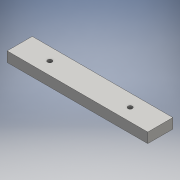
# Autodesk Inventor part: xyStagePostAttach
Saved by Autodesk Inventor 2016 (Build 200138000, 138)
## iProperties
Created: 2016-09-30
Part Number: xyStagePostAttach
Material: Generic
Document SubType Name: Modeling
Designer: sims01
Density: 1 g/cm^3
Appearance: Default
Author: sims01
Autodesk Inventor part; units mm, degrees
ref_plane "YZ Plane" through (0, 0, 0) normal (1, 0, 0) x (0, 1, 0)
ref_plane "XZ Plane" through (0, 0, 0) normal (0, 1, 0) x (-1, 0, 0)
ref_plane "XY Plane" through (0, 0, 0) normal (0, 0, 1) x (1, 0, 0)
sketch "Sketch1" plane through (0, 0, 0) normal (0, 0, 1) x (1, 0, 0)
  line L0 (-70, 12.5) -> (70, 12.5)
  line L1 (70, 12.5) -> (70, -12.5)
  line L2 (70, -12.5) -> (-70, -12.5)
  line L3 (-70, -12.5) -> (-70, 12.5)
  point P0 (0, 0)
  dimension "d0" = 140
  dimension "d1" = 25
  dimension "d2" = 70
  dimension "d3" = 12.5
  constraints: 8 end point, 2 parallel, 1 horizontal, 1 perpendicular
  measures "d0" distance of L0.start L0.end
  measures "d1" distance of L0.end L1.end
  measures "d2" distance from line of point (0, 0) L1
  measures "d3" distance from line of point (0, 0) L0
extrude "Extrusion1" add sketch "Sketch1" along normal blind 10
sketch "Sketch2" plane through (0, 0, 10) normal (0, 0, 1) x (1, 0, 0)
  point P0 (0, 0)
  point P1 (-40, 0)
  point P2 (40, 0)
  dimension "d6" = 80
  dimension "d7" = 40
  constraints: 2 horizontal alignment
  measures "d6" distance of point (-40, 0) point (40, 0)
  measures "d7" distance of point (40, 0) point (0, 0)
hole "Hole1" at (-40, 0, 10) at (40, 0, 10) direction (0, 0, -1) diameter 4.5 end through all clearance for "Countersunk Flat Head Screw ISO 2009/7046" size "M4" standard "ISO"
equation "\"d2\" = 0.5 * d0"
equation "\"d3\" = 0.5 * d1"
equation "\"d7\" = 0.5 * d6"
body "Solid1"
